Autodesk Fusion 360 part; units mm, degrees
note: some values were not read from the file. Set by a fixed rule: which face or edge a step refers to.
(part 3 of 3)
equation "d52 = JoinSize"
equation "d53 = JoinLenght"
equation "d54 = JoinSize"
equation "d55 = JoinLenght"
equation "d56 = JoinSize"
equation "d57 = JoinLenght"
equation "d58 = JoinSize"
equation "d59 = JoinLenght"
equation "d60 = JoinSize"
equation "d61 = JoinLenght"
equation "d62 = JoinSize"
equation "d63 = JoinLenght"
equation "d64 = JoinSize"
equation "d65 = JoinLenght"
equation "d66 = JoinSize"
equation "d69 = -RequiredPinDepth - 1 mm"
equation "d71 = DownTunnelDepth"
equation "d75 = -WoodHeight"
equation "d78 = -WoodHeight"
equation "d84 = -RequiredPinDepth + 0.5 mm"
equation "d88 = ClassicBitMarge"
equation "d89 = -WoodHeight"
equation "RequiredPinDepth = WoodHeight - PinHeight - 2 mm"
equation "d108 = ClassicBitMarge"
equation "d109 = ClassicBitMarge"
equation "d110 = ClassicBitMarge"
equation "d111 = ClassicBitMarge"
equation "d113 = ClassicBitMarge"
equation "d114 = ClassicBitMarge"
equation "d115 = -WoodHeight"
equation "d139 = DownTunnelDepth"
equation "d143 = -WoodHeight"
equation "d144 = -RequiredPinDepth - 1 mm"
equation "d155 = -RequiredPinDepth - 1 mm"
equation "d157 = DownTunnelDepth"
equation "d161 = -WoodHeight"
equation "d171 = -WoodHeight"
equation "DownTunnelDepth = 4 mm"
equation "d174 = -WoodHeight"
equation "d180 = -WoodHeight"
equation "d182 = -WoodHeight"
equation "d184 = -WoodHeight"
named bodies: "WoodBoard", "WoodBoard Down"
